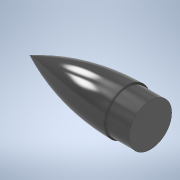
# Autodesk Inventor part: Nose
Saved by Autodesk Inventor 2020 (Build 240168000, 168)
## iProperties
Created: 2022-11-08
Part Number: Nose
Material: PLA
Document SubType Name: Modeling
Designer: Hp
Density: 1.3 g/cm^3
Appearance: Dark Gray
Author: Hp
Autodesk Inventor part; units mm, degrees
ref_plane "YZ Plane" through (0, 0, 0) normal (1, 0, 0) x (0, 1, 0)
ref_plane "XZ Plane" through (0, 0, 0) normal (0, 1, 0) x (-1, 0, 0)
ref_plane "XY Plane" through (0, 0, 0) normal (0, 0, 1) x (1, 0, 0)
sketch "Sketch1" plane through (0, 0, 0) normal (0, 0, 1) x (1, 0, 0)
  line L0 (0, 0) -> (170, 0)
  line L1 (170, 35) -> (170, 39.5)
  arc A0 (170, 39.5) -> (0, 0) centre (170, -346.0728) ccw
  line L2 (170, 0) -> (210, 0)
  line L3 (210, 0) -> (210, 37)
  line L4 (210, 37) -> (170, 37)
  line L5 (170, 37) -> (170, 35)
  arc A1 (168, 37.4948) -> (8.8373, 2) centre (170, -346.0728) ccw
  line L6 (168, 37.4948) -> (170, 37.4948)
  line L7 (8.8373, 2) -> (4.5862, 0)
  line L8 (172, 35) -> (208, 35)
  line L9 (208, 35) -> (208, 2)
  line L10 (172, 35) -> (170, 35)
  line L11 (208, 2) -> (208, 0)
  dimension "d1" = 39.5
  dimension "d2" = 40
  dimension "d3" = 37
  dimension "d4" = 2
  dimension "d5" = 2
  constraints: 24 end point, 5 perpendicular, 4 point on circle, 3 point on line, 2 centre point, 2 horizontal, 2 parallel, 1 other
  measures "d1" distance of L1.end L0.end
  measures "d2" distance of L4.end L3.end
  measures "d3" distance of L3.end L2.end
  measures "d4" radial gap between concentric circles of A0 A1
  measures "d5" distance between parallel lines of L4 L8
revolve "Revolution1" add sketch "Sketch1" angle 360 about axis through (0, 0, 0) along (1, 0, 0) contours A0 L1 L6 A1 L7 L0 | L11 L9 L8 L10 L1 L4 L3 L2
body "Solid1"
